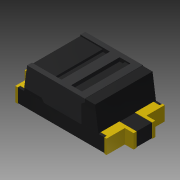
# Autodesk Inventor part: GP2S60
Saved by Autodesk Inventor 2015 (Build 190159000, 159)
## iProperties
Created: 2015-11-23
Part Number: GP2S60
Material: Generic
Document SubType Name: Modeling
Designer: Danil
Density: 1 g/cm^3
Appearance: Default
Author: Danil
Autodesk Inventor part; units mm, degrees
ref_plane "YZ Plane" through (0, 0, 0) normal (1, 0, 0) x (0, 1, 0)
ref_plane "XZ Plane" through (0, 0, 0) normal (0, 1, 0) x (-1, 0, 0)
ref_plane "XY Plane" through (0, 0, 0) normal (0, 0, 1) x (1, 0, 0)
sketch "Sketch1" plane through (0, 0, 0) normal (0, 0, 1) x (1, 0, 0)
  line L0 (1.35, -0.85) -> (-1.35, -0.85)
  line L1 (-1.35, -0.85) -> (-1.35, 0.85)
  line L2 (-1.35, 0.85) -> (1.35, 0.85)
  line L3 (1.35, 0.85) -> (1.35, -0.85)
  line L4 (1.35, -0.85) -> (-1.35, 0.85) construction
  line L5 (-1.35, -0.85) -> (1.35, 0.85) construction
  line L6 (-1.35, 0) -> (1.35, 0) construction
  line L7 (0, 0.85) -> (0, -0.85) construction
  line L8 (1.6, -0.32) -> (1.35, -0.32)
  line L9 (1.35, -0.32) -> (1.35, 0.32)
  line L10 (1.35, 0.32) -> (1.6, 0.32)
  line L11 (1.6, 0.32) -> (1.6, -0.32)
  line L12 (1.6, -0.32) -> (1.35, 0.32) construction
  line L13 (1.35, -0.32) -> (1.6, 0.32) construction
  line L14 (-1.6, -0.32) -> (-1.35, -0.32)
  line L15 (-1.35, -0.32) -> (-1.35, 0.32)
  line L16 (-1.35, 0.32) -> (-1.6, 0.32)
  line L17 (-1.6, 0.32) -> (-1.6, -0.32)
  line L18 (-1.6, -0.32) -> (-1.35, 0.32) construction
  line L19 (-1.35, -0.32) -> (-1.6, 0.32) construction
  point P0 (0, 0)
  point P1 (1.475, 0)
  point P2 (-1.475, 0)
  dimension "d0" = 2.7
  dimension "d1" = 1.7
  dimension "d3" = 0.64
  dimension "d4" = 3.2
  constraints: 40 end point, 10 midpoint, 5 symmetric about line, 4 parallel, 3 perpendicular, 1 collinear, 1 horizontal, 1 point on line
  measures "d0" distance of L1.end L2.end
  measures "d1" distance of L0.end L1.end
  measures "d3" distance of L10.end L8.start
  measures "d4" distance between parallel lines of L11 L17
extrude "Extrusion1" add sketch "Sketch1" along normal blind 0.4
sketch "Sketch2" plane through (0, 0, 0.4) normal (0, 0, 1) x (1, 0, 0)
  line L0 (-1.1, -0.8495) -> (1.1, -0.8495)
  line L1 (1.1, -0.8495) -> (1.1, 0.8495)
  line L2 (1.1, 0.8495) -> (-1.1, 0.8495)
  line L3 (-1.1, 0.8495) -> (-1.1, -0.8495)
  line L4 (-1.1, -0.8495) -> (1.1, 0.8495) construction
  line L5 (1.1, -0.8495) -> (-1.1, 0.8495) construction
  point P0 (0, 0)
  dimension "d7" = 2.2
  dimension "d27" = 1.699
  constraints: 12 end point, 2 midpoint, 2 parallel, 1 horizontal, 1 perpendicular
  measures "d7" distance of L2.end L1.end
  measures "d27" distance of L0.end L1.end
sketch "Sketch3" plane through (0, 0, 0) normal (0, 0, -1) x (-1, 0, 0)
  line L0 (1.35, -0.85) -> (-1.35, -0.85) projected
  line L1 (-0.9, 0.85) -> (0.9, 0.85)
  line L2 (0.9, 0.85) -> (0.9, -0.85)
  line L3 (0.9, -0.85) -> (-0.9, -0.85)
  line L4 (-0.9, -0.85) -> (-0.9, 0.85)
  line L5 (-0.9, 0.85) -> (0.9, -0.85) construction
  line L6 (0.9, 0.85) -> (-0.9, -0.85) construction
  line L7 (1.28, 0.85) -> (-1.28, 0.85)
  line L8 (-1.28, 0.85) -> (-1.28, 0.78)
  line L9 (-1.28, 0.78) -> (1.28, 0.78)
  line L10 (1.28, 0.78) -> (1.28, 0.85)
  line L11 (1.28, 0.85) -> (-1.28, 0.78) construction
  line L12 (-1.28, 0.85) -> (1.28, 0.78) construction
  line L13 (-1.35, 0.85) -> (-1.35, 0.32) projected
  line L14 (-1.6, -0.32) -> (-1.6, 0.32) projected
  line L15 (1.6, 0.23) -> (-1.6, 0.23)
  line L16 (-1.6, 0.23) -> (-1.6, -0.23)
  line L17 (-1.6, -0.23) -> (1.6, -0.23)
  line L18 (1.6, -0.23) -> (1.6, 0.23)
  line L19 (1.6, 0.23) -> (-1.6, -0.23) construction
  line L20 (-1.6, 0.23) -> (1.6, -0.23) construction
  line L21 (1.35, -0.85) -> (1.35, -0.32)
  line L22 (1.35, -0.32) -> (1.6, -0.32)
  line L23 (1.6, -0.32) -> (1.35, -0.32) projected
  line L24 (1.6, -0.32) -> (1.6, 0.32)
  line L25 (1.6, 0.32) -> (1.35, 0.32)
  line L26 (1.35, 0.32) -> (1.35, 0.85)
  line L27 (-1.35, 0.85) -> (1.35, 0.85) projected
  line L28 (1.35, 0.85) -> (-1.35, 0.85)
  line L29 (-1.35, 0.85) -> (-1.35, 0.32)
  line L30 (-1.35, 0.32) -> (-1.6, 0.32)
  line L31 (-1.6, 0.32) -> (-1.35, 0.32) projected
  line L32 (-1.6, -0.32) -> (-1.35, -0.32)
  line L33 (-1.35, -0.32) -> (-1.6, -0.32) projected
  line L34 (-1.35, -0.32) -> (-1.35, -0.85)
  line L35 (1.6, 0) -> (-1.6, 0) construction
  line L36 (-0.9, -0.85) -> (0.9, -0.85)
  line L37 (-0.9, -0.85) -> (0.9, 0.85) construction
  line L38 (0.9, -0.85) -> (-0.9, 0.85) construction
  line L39 (1.28, -0.85) -> (-1.28, -0.85)
  line L40 (-1.28, -0.85) -> (-1.28, -0.78)
  line L41 (-1.28, -0.78) -> (1.28, -0.78)
  line L42 (1.28, -0.78) -> (1.28, -0.85)
  line L43 (1.28, -0.85) -> (-1.28, -0.78) construction
  line L44 (-1.28, -0.85) -> (1.28, -0.78) construction
  line L45 (1.35, -0.85) -> (-1.35, -0.85)
  line L46 (-0.3, -0.18) -> (0.3, -0.18)
  line L47 (0.3, -0.18) -> (0.3, -0.78)
  line L48 (0.3, -0.78) -> (-0.3, -0.78)
  line L49 (-0.3, -0.78) -> (-0.3, -0.18)
  line L50 (-0.3, -0.18) -> (0.3, -0.78) construction
  line L51 (0.3, -0.18) -> (-0.3, -0.78) construction
  circle A0 centre (0, 0.48) radius 0.3
  circle A1 centre (0, 0.48) radius 0.2
  line L52 (0.05, -0.18) -> (0.05, 0.1842)
  line L53 (-0.05, 0.1842) -> (-0.05, -0.18)
  line L54 (0, -0.85) -> (0, 0.85) construction
  circle A2 centre (0, -0.48) radius 0.2
  point P0 (0, 0)
  point P1 (0, 0.815)
  point P2 (0, 0.815)
  point P3 (0, 0)
  point P4 (0, -0.815)
  point P5 (0, -0.815)
  point P6 (0, -0.48)
  point P7 (0, -0.48)
  point P8 (0, 0)
  point P9 (0, -0.48)
  point P10 (0, 0)
  dimension "d8" = 1.8
  dimension "d9" = 0.07
  dimension "d10" = 0.07
  dimension "d11" = 0.46
  dimension "d14" = 0.6
  dimension "d15" = 0.6
  dimension "d16" = 0.4
  dimension "d17" = 0.1
  dimension "d18" = 0.4
  constraints: 96 end point, 21 midpoint, 12 equal length, 12 perpendicular, 10 symmetric about line, 6 point on line, 4 horizontal, 3 centre point, 3 vertical alignment, 2 collinear, 2 point on circle, 1 coincident, 1 tangent, 1 vertical, 1 other
  measures "d8" distance of L2.end L3.end
  measures "d9" distance of L7.end L8.end
  measures "d10" distance between parallel lines of L13 L8
  measures "d11" distance between parallel lines of L15 L17
  measures "d14" distance of L48.end L46.start
  measures "d15" diameter of A0
  measures "d16" diameter of A1
  measures "d17" distance between parallel lines of L52 L53
  measures "d18" diameter of A2
extrude "Extrusion2" add sketch "Sketch3" along normal blind 0.01 contours L0 L42 L41 L2 L17 L24 L22 L21 | L0 L34 L32 L14 L17 L4 L41 L40 | L41 L49 L17 L47 | L15 L2 L9 L10 L27 L26 L25 L24 | L17 L49 L46 L47 | L15 L14 L30 L13 L27 L8 L9 L4 | A0 L15 | L15 A0 | L52 L46 L53 A0
extrude "Extrusion3" add sketch "Sketch2" along normal blind 0.7
chamfer "Chamfer1" distance 0.1 distance2 0.7 1 edges at (-1.1, 0, 1.1) measured on face at (-0.3667, 0.2832, 1.1)
chamfer "Chamfer2" distance 0.1 distance2 0.7 1 edges at (1.1, 0, 1.1) measured on face at (-0.3003, 0.2832, 1.1)
sketch "Sketch5" plane through (0, 0, 0.4) normal (0, 0, 1) x (1, 0, 0)
  line L0 (-0.9, 0.85) -> (0.9, 0.85)
  line L1 (0.9, 0.85) -> (0.9, -0.85)
  line L2 (0.9, -0.85) -> (-0.9, -0.85)
  line L3 (-0.9, -0.85) -> (-0.9, 0.85)
  line L4 (-0.9, 0.85) -> (0.9, -0.85) construction
  line L5 (0.9, 0.85) -> (-0.9, -0.85) construction
  line L6 (1.28, 0.85) -> (-1.28, 0.85)
  line L7 (-1.28, 0.85) -> (-1.28, 0.78)
  line L8 (-1.28, 0.78) -> (1.28, 0.78)
  line L9 (1.28, 0.78) -> (1.28, 0.85)
  line L10 (1.28, 0.85) -> (-1.28, 0.78) construction
  line L11 (-1.28, 0.85) -> (1.28, 0.78) construction
  line L12 (1.6, 0.23) -> (-1.6, 0.23)
  line L13 (-1.6, 0.23) -> (-1.6, -0.23)
  line L14 (-1.6, -0.23) -> (1.6, -0.23)
  line L15 (1.6, -0.23) -> (1.6, 0.23)
  line L16 (1.6, 0.23) -> (-1.6, -0.23) construction
  line L17 (-1.6, 0.23) -> (1.6, -0.23) construction
  line L18 (1.35, -0.85) -> (1.35, -0.32)
  line L19 (1.35, -0.32) -> (1.6, -0.32)
  line L20 (1.6, -0.32) -> (1.6, 0.32)
  line L21 (1.6, 0.32) -> (1.35, 0.32)
  line L22 (1.35, 0.32) -> (1.35, 0.85)
  line L23 (1.35, 0.85) -> (-1.35, 0.85)
  line L24 (-1.35, 0.85) -> (-1.35, 0.32)
  line L25 (-1.35, 0.32) -> (-1.6, 0.32)
  line L26 (-1.6, -0.32) -> (-1.35, -0.32)
  line L27 (-1.35, -0.32) -> (-1.35, -0.85)
  line L28 (1.6, 0) -> (-1.6, 0) construction
  line L29 (-1.28, -0.85) -> (-1.28, -0.78)
  line L30 (-0.9, -0.85) -> (0.9, -0.85)
  line L31 (-0.9, -0.85) -> (0.9, 0.85) construction
  line L32 (0.9, -0.85) -> (-0.9, 0.85) construction
  line L33 (1.35, -0.85) -> (-1.35, -0.85)
  line L34 (1.28, -0.85) -> (-1.28, -0.85)
  line L35 (-1.28, -0.78) -> (1.28, -0.78)
  line L36 (1.28, -0.85) -> (-1.28, -0.78) construction
  line L37 (-1.28, -0.85) -> (1.28, -0.78) construction
  line L38 (1.28, -0.78) -> (1.28, -0.85)
  line L39 (-0.3, -0.18) -> (0.3, -0.18)
  line L40 (0.3, -0.18) -> (0.3, -0.78)
  line L41 (0.3, -0.78) -> (-0.3, -0.78)
  line L42 (-0.3, -0.78) -> (-0.3, -0.18)
  line L43 (-0.3, -0.18) -> (0.3, -0.78) construction
  line L44 (0.3, -0.18) -> (-0.3, -0.78) construction
  circle A0 centre (0, 0.48) radius 0.3
  circle A1 centre (0, 0.48) radius 0.2
  line L45 (0.05, -0.18) -> (0.05, 0.1842)
  line L46 (-0.05, 0.1842) -> (-0.05, -0.18)
  line L47 (0, -0.85) -> (0, 0.85) construction
  circle A2 centre (0, -0.48) radius 0.2
  line L48 (-1.6, 0.32) -> (-1.6, -0.32)
  line L49 (-1.35, 0.32) -> (-1.6, 0.32) projected
  point P0 (0, 0)
  point P1 (0, 0.815)
  point P2 (0, 0.815)
  point P3 (0, 0)
  point P4 (0, -0.815)
  point P5 (0, -0.815)
  point P6 (0, -0.48)
  point P7 (0, -0.48)
  point P8 (0, 0)
  point P9 (0, -0.48)
  point P10 (0, 0)
  dimension "d30" = 1.8
  dimension "d31" = 0.07
  dimension "d33" = 0.46
  dimension "d34" = 0.6
  dimension "d35" = 0.6
  dimension "d36" = 0.4
  dimension "d37" = 0.1
  dimension "d38" = 0.4
  constraints: 98 end point, 21 midpoint, 11 perpendicular, 10 symmetric about line, 8 parallel, 4 horizontal, 4 point on line, 3 centre point, 3 vertical alignment, 2 collinear, 2 point on circle, 1 coincident, 1 tangent, 1 vertical, 1 other
  measures "d30" distance of L1.end L2.end
  measures "d31" distance of L6.end L7.end
  measures "d33" distance between parallel lines of L12 L14
  measures "d34" distance of L41.end L39.start
  measures "d35" diameter of A0
  measures "d36" diameter of A1
  measures "d37" distance between parallel lines of L45 L46
  measures "d38" diameter of A2
extrude "Extrusion5" add sketch "Sketch5" along normal blind 0.01 contours L3 L12 L48 L25 L24 L23 L7 L8 | L8 L9 L23 L22 L21 L20 L12 L1 | L3 L35 L29 L33 L27 L26 L48 L14 | L14 L20 L19 L18 L33 L38 L35 L1
sketch "Sketch6" plane through (-1.28, 0.85, 0) normal (0, 1, 0) x (1, 0, 0)
  line L0 (0, 0.01) -> (-0.07, 0.01)
  line L1 (-0.07, 0.01) -> (-0.07, -0.41)
  line L2 (-0.07, -0.41) -> (0, -0.41)
  line L3 (0, -0.41) -> (0, 0.01)
  line L4 (2.3786, -0.41) -> (2.88, -0.41) projected
  line L5 (2.56, 0.01) -> (2.6293, 0.01)
  line L6 (2.6293, 0.01) -> (2.6293, -0.41)
  line L7 (2.6293, -0.41) -> (2.56, -0.41)
  line L8 (2.56, -0.41) -> (2.56, 0.01)
  point P0 (1.28, 0)
  constraints: 16 end point, 4 parallel, 2 horizontal, 2 perpendicular, 1 midpoint
extrude "Extrusion6" add sketch "Sketch6" along normal blind 0.01
sketch "Sketch7" plane through (-1.28, -0.85, 0) normal (0, -1, 0) x (1, 0, 0)
  line L0 (0, -0.01) -> (-0.07, -0.01)
  line L1 (-0.07, -0.01) -> (-0.07, 0.41)
  line L2 (-0.07, 0.41) -> (0, 0.41)
  line L3 (0, 0.41) -> (0, -0.01)
  line L4 (2.63, -0.01) -> (2.56, -0.01)
  line L5 (2.56, -0.01) -> (2.56, 0.41)
  line L6 (2.56, 0.41) -> (2.63, 0.41)
  line L7 (2.63, 0.41) -> (2.63, -0.01)
  point P0 (1.28, 0)
  constraints: 16 end point, 4 parallel, 2 horizontal, 2 perpendicular, 1 point on line
extrude "Extrusion7" add sketch "Sketch7" along normal blind 0.01
sketch "Sketch8" plane through (1.6, -0.23, 0) normal (1, 0, 0) x (0, 0, -1)
  line L0 (-0.41, -0.09) -> (0.01, -0.09)
  line L1 (0.01, -0.09) -> (0.01, 0)
  line L2 (0.01, 0) -> (-0.41, 0)
  line L3 (-0.41, 0) -> (-0.41, -0.09)
  line L4 (0.01, 0.55) -> (-0.41, 0.55)
  line L5 (-0.41, 0.55) -> (-0.41, 0.46)
  line L6 (-0.41, 0.46) -> (0.01, 0.46)
  line L7 (0.01, 0.46) -> (0.01, 0.55)
  point P0 (0, 0.23)
  constraints: 16 end point, 4 parallel, 2 horizontal, 2 perpendicular
extrude "Extrusion8" add sketch "Sketch8" along normal blind 0.01
sketch "Sketch9" plane through (-1.6, -0.23, 0) normal (-1, 0, 0) x (0, 0, 1)
  line L0 (-0.01, -0.09) -> (0.41, -0.09)
  line L1 (0.41, -0.09) -> (0.41, 0)
  line L2 (0.41, 0) -> (-0.01, 0)
  line L3 (-0.01, 0) -> (-0.01, -0.09)
  line L4 (0.41, 0.46) -> (-0.01, 0.46)
  line L5 (-0.01, 0.46) -> (-0.01, 0.55)
  line L6 (-0.01, 0.55) -> (0.41, 0.55)
  line L7 (0.41, 0.55) -> (0.41, 0.46)
  point P0 (0, 0.23)
  constraints: 16 end point, 4 parallel, 2 horizontal, 2 perpendicular
extrude "Extrusion9" add sketch "Sketch9" along normal blind 0.01
sketch "Sketch10" plane through (0, 0, 1.1) normal (0, 0, 1) x (1, 0, 0)
  line L0 (0.48, 0.7171) -> (0.1599, 0.7171)
  line L1 (0.1599, 0.7171) -> (0.1599, -0.7171)
  line L2 (0.1599, -0.7171) -> (0.48, -0.7171)
  line L3 (0.48, -0.7171) -> (0.48, 0.7171)
  line L4 (0.48, 0.7171) -> (0.1599, -0.7171) construction
  line L5 (0.1599, 0.7171) -> (0.48, -0.7171) construction
  line L6 (-1.0459, 0.7171) -> (-0.1265, 0.7171)
  line L7 (-0.1265, 0.7171) -> (-0.1265, -0.7171)
  line L8 (-0.1265, -0.7171) -> (-1.0459, -0.7171)
  line L9 (-1.0459, -0.7171) -> (-1.0459, 0.7171)
  line L10 (-1.0459, 0.7171) -> (-0.1265, -0.7171) construction
  line L11 (-0.1265, 0.7171) -> (-1.0459, -0.7171) construction
  line L12 (0.1599, -0.7171) -> (0.3199, -0.7171)
  line L13 (0.3199, -0.7171) -> (0.3199, 0.7171)
  line L14 (0.3199, 0.7171) -> (0.1599, 0.7171)
  line L15 (0.1599, 0.7171) -> (0.1599, -0.7171)
  line L16 (-0.1265, -0.7171) -> (-0.3365, -0.7171)
  line L17 (-0.3365, -0.7171) -> (-0.3365, 0.7171)
  line L18 (-0.3365, 0.7171) -> (-0.1265, 0.7171)
  line L19 (-0.1265, 0.7171) -> (-0.1265, -0.7171)
  line L20 (-1, -0.8495) -> (-1, 0.8495) projected
  point P0 (0, 0)
  point P1 (0.3199, 0)
  point P2 (-0.5862, 0)
  point P3 (-0.5862, 0)
  point P4 (0.3199, 0)
  point P5 (-0.5862, 0)
  constraints: 40 end point, 8 midpoint, 8 parallel, 4 horizontal, 4 perpendicular, 3 horizontal alignment, 2 point on line
extrude "Extrusion10" cut sketch "Sketch10" against normal blind 0.1 contours L13 L2 L1 L0 | L6 L7 L8 L17
extrude "Extrusion11" cut sketch "Sketch10" against normal blind 0.03 contours L3 L2 L13 L0 | L17 L8 L20 L6 | L20 L8 L9 L6
sketch "Sketch11" plane through (0, 0, 1.1) normal (0, 0, 1) x (1, 0, 0)
  line L0 (-1, -0.8495) -> (1, -0.8495) projected
  line L1 (0.703, -0.8495) -> (-1, -0.8495)
  line L2 (-1, -0.8495) -> (-1, 0.8495)
  line L3 (-1, 0.8495) -> (0.703, 0.8495)
  line L4 (0.703, 0.8495) -> (0.703, -0.8495)
  line L5 (0.48, -0.7171) -> (0.1599, -0.7171)
  line L6 (0.1599, -0.7171) -> (0.1599, 0.7171)
  line L7 (0.1599, 0.7171) -> (0.48, 0.7171)
  line L8 (0.48, 0.7171) -> (0.48, -0.7171)
  line L9 (-0.1271, -0.7171) -> (-1, -0.7171)
  line L10 (-1, -0.7171) -> (-1, 0.7171)
  line L11 (-1, 0.7171) -> (-0.1271, 0.7171)
  line L12 (-0.1271, 0.7171) -> (-0.1271, -0.7171)
  point P0 (0, 0)
  constraints: 24 end point, 6 parallel, 3 horizontal, 3 perpendicular, 2 point on line
extrude "Extrusion12" add sketch "Sketch11" along normal blind 0.01 contours L2 L9 L12 L11 L3 L4 L0
sketch "Sketch12" plane through (-1.1, 0.8495, 0.4) normal (0, 1, 0) x (1, 0, 0)
  line L0 (1.803, -0.7) -> (1.803, -0.613)
  line L1 (1.803, -0.613) -> (1.6921, -0.5249)
  line L2 (1.6921, -0.5249) -> (1.6921, -0.005)
  line L3 (1.6921, -0.005) -> (0.5959, -0.005)
  line L4 (0.5959, -0.005) -> (0.5238, -0.0957)
  line L5 (0.5238, -0.0957) -> (0.0137, -0.0957)
  line L6 (0.1, -0.7) -> (0, 0) projected
  line L7 (1.803, -0.71) -> (1.803, -0.7)
  line L8 (1.803, -0.7) -> (1.803, -0.71) projected
  line L9 (0.1, -0.71) -> (0.1, -0.7)
  line L10 (0.1, -0.7) -> (0.0137, -0.0957)
  line L11 (0, 0) -> (0.1, -0.7) projected
  line L12 (1.803, -0.71) -> (0.1, -0.71)
  line L13 (0.1, -0.71) -> (1.803, -0.71) projected
  point P0 (1.1, 0.4)
  constraints: 20 end point, 3 collinear, 2 parallel, 2 perpendicular, 2 vertical, 1 point on line
extrude "Extrusion13" add sketch "Sketch12" along normal blind 0.01
sketch "Sketch13" plane through (-1.1, -0.8495, 0.4) normal (0, -1, 0) x (1, 0, 0)
  line L0 (0.0137, 0.0957) -> (0.1, 0.7)
  line L1 (0.0137, 0.0957) -> (0.1, 0.7) projected
  line L2 (0.1, 0.7) -> (0.1, 0.71)
  line L3 (0.1, 0.71) -> (0.9729, 0.71) projected
  line L4 (0.1, 0.71) -> (1.803, 0.71)
  line L5 (2.1, 0.7) -> (1.803, 0.7) projected
  line L6 (1.803, 0.71) -> (1.803, 0.7)
  line L7 (1.803, 0.7) -> (1.803, 0.613)
  line L8 (1.803, 0.613) -> (1.6921, 0.5249)
  line L9 (1.6921, 0.5249) -> (1.803, 0.613) projected
  line L10 (1.6921, 0.5249) -> (1.6921, 0)
  line L11 (2.2, 0) -> (0, 0) projected
  line L12 (0.0137, 0.0957) -> (0.5238, 0.0957)
  line L13 (0.5238, 0.0957) -> (0.5999, 0)
  line L14 (1.6921, 0) -> (0.5999, 0)
  constraints: 20 end point, 3 collinear, 3 parallel, 3 perpendicular, 2 point on line, 1 horizontal
extrude "Extrusion14" add sketch "Sketch13" along normal blind 0.01
body "Solid1"
